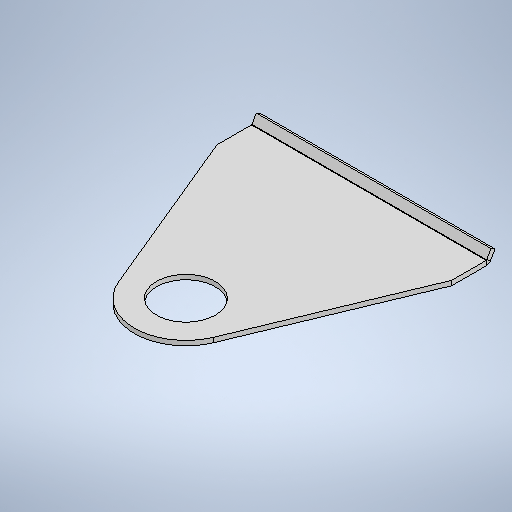
# Autodesk Inventor part: NVPH-301 back side
Saved by Autodesk Inventor 2025.1 (Build 291241020, 241B)
## iProperties
Created: 2024-12-03
Part Number: NVPH-301 back side
Material: Generic
Document SubType Name: Sheet Metal
Designer: user
Density: 1 g/cm^3
Sheet Metal Rule: Default
Appearance: Default
Flat Pattern Width: 52.4063 cm
Flat Pattern Length: 50 cm
Flat Pattern Area: 2620.31 cm^2
Sheet Metal Width: 524.063 mm
Sheet Metal Length: 500.000 mm
Sheet Metal Area: 262031.350 mm^2
Author: user
Autodesk Inventor part; units mm, degrees
ref_plane "YZ Plane" through (0, 0, 0) normal (1, 0, 0) x (0, 1, 0)
ref_plane "XZ Plane" through (0, 0, 0) normal (0, 1, 0) x (-1, 0, 0)
ref_plane "XY Plane" through (0, 0, 0) normal (0, 0, 1) x (1, 0, 0)
sketch "Sketch1" plane through (0, 0, 0) normal (0, 0, 1) x (1, 0, 0)
  line L0 (0, 0) -> (0, 506.1095)
  line L1 (-250, 506.1095) -> (250, 506.1095)
  circle A0 centre (0, 110) radius 62.5
  circle A1 centre (0, 110) radius 110
  line L2 (-250, 506.1095) -> (-250, 426.1095)
  line L3 (-250, 426.1095) -> (-101.6267, 67.9048)
  line L4 (250, 506.1095) -> (250, 426.1095)
  line L5 (250, 426.1095) -> (101.6267, 67.9048)
  dimension "d0" = 506.1095
  dimension "d1" = 500
  dimension "d2" = 125
  dimension "d4" = 80
  dimension "d16" = 45
  dimension "d17" = 220
  measures "d0" distance of L0.end L0.start
  measures "d1" distance of L1.start L1.end
  measures "d2" diameter of A0
  measures "d4" distance of L1.start L2.end
  measures "d16" angle of L5 L3
  measures "d17" diameter of A1
extrude "Plate1" add sketch "Sketch1" along normal blind 10 contours A1 L0 A0 | L0 A0 A1 | L3 L2 L1 L0 A1 | A1 L0 L1 L4 L5
sketch "Sketch2" plane through (-250, 497.4493, 5) normal (0, 0.8660254, -0.5) x (-1, 0, 0)
  line L0 (-500, 0) -> (0, 0)
  line L1 (0, 0) -> (0, 25)
  line L2 (0, 25) -> (-500, 25)
  line L3 (-500, 25) -> (-500, 0)
  constraints: 6 end point, 1 horizontal, 1 perpendicular, 1 vertical
edge flange "Flange1" height 25 angle 60 thickness 10 bend radius 1 thickness toward (0, 0.8660254, -0.5) relief straight relief width 10 relief depth 5 edges at (0, 506.1095, 10) wall of the first edge with corners at (250, 497.4493, 5) (-250, 497.4493, 5) (-250, 509.9493, 26.6506) (250, 509.9493, 26.6506)
bend "Bend1"
corner "Corner1"
equation "\"d2\" = back_steel_circle_проходной_диаметр"
equation "\"d5\" = Thickness"
equation "\"d6\" = BendReliefWidth"
equation "\"d7\" = BendReliefDepth"
equation "\"d8\" = MinimumRemnant"
equation "\"d9\" = TransitionRadius"
equation "\"d13\" = CornerReliefSize"
equation "\"d14\" = GapSize"
equation "\"d15\" = JacobiRadiusSize"
equation "\"BendReliefDepth\" = 0.5 * Thickness"
equation "\"back_steel_circle_проходной_диаметр\" = 125"
equation "\"Thickness\" = 10"
equation "\"BendReliefWidth\" = 10"
equation "\"MinimumRemnant\" = 20"
equation "\"TransitionRadius\" = 10"
equation "\"CornerReliefSize\" = 40"
equation "\"GapSize\" = 10"
equation "\"JacobiRadiusSize\" = 10"
body "Solid1"
